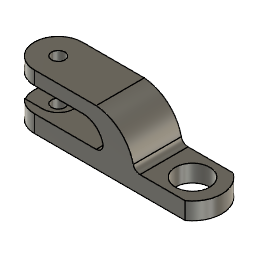
11_largage_moteur_manivelle (Autodesk Fusion 360 design; units mm, degrees)
Autodesk Fusion 360 part; units mm, degrees
note: some values were not read from the file. Set by a fixed rule: which sketch regions a step uses.
sketch "Esquisse2" plane through (0, 0, 0) normal (0, 0, 1) x (1, 0, 0)
  line L0 (0, 0) -> (34.1782, 0)
  line L1 (0, 14) -> (34.1782, 14)
  arc A0 (0, 14) -> (0, 0) centre (0, 7) ccw
  circle A1 centre (0, 7) radius 1.95
  circle A2 centre (39, 7) radius 5
  line L2 (39, 7) -> (46, 7) construction
  arc A3 (43.8218, 0) -> (43.8218, 14) centre (39, 7) ccw
  line L3 (34.1782, 14) -> (43.8218, 14)
  line L4 (34.1782, 0) -> (43.8218, 0)
  dimension "d10" = 3.9
  dimension "d15" = 17
  dimension "d16" = 39
  dimension "d17" = 10
  dimension "d18" = 14
  constraint coincident L0.start A0.end
  constraint horizontal L0
  constraint tangent L1 A0
  constraint tangent L0 A0
  constraint concentric A0 A1
  constraint coincident A2.centre L2.start
  constraint concentric A2 A3
  constraint parallel L1 L3
  constraint parallel L0 L4
  measures "d10" diameter of A1
  measures "d15" diameter of A3
  measures "d16" distance of A0.centre A2.centre
  measures "d17" diameter of A2
  measures "d18" distance of L0 L1
extrude "Extrusion1" add sketch "Esquisse2" along normal blind 16
sketch "Esquisse3" plane through (0, 0, 0) normal (0, 1, 0) x (1, 0, 0)
  line L0 (-7, 0) -> (-7, -5) construction
  line L1 (-7, -16.0714) -> (-7, -12.0714) construction
  line L2 (-7, -12.0714) -> (14.0533, -12.0714)
  arc A0 (18, -16) -> (28.7636, -6.5727) centre (17, -4) ccw
  line L3 (30.7174, -5) -> (48, -5)
  line L4 (48, -5) -> (48, -16)
  line L5 (18, -16) -> (48, -16)
  arc A1 (30.7174, -5) -> (28.7636, -6.5727) centre (30.7174, -7) ccw
  line L6 (18, -5) -> (-7, -5)
  line L7 (-7, -12.0714) -> (-7, -5)
  arc A2 (19.9387, -7.4912) -> (18, -5) centre (18, -7) ccw
  arc A3 (14.0533, -12.0714) -> (19.9387, -7.4912) centre (14.0533, -6) ccw
  point P0 (18, -12.0714)
  dimension "d21" = 5
  dimension "d22" = 4
  dimension "d23" = 25
  dimension "d25" = 2
  constraint vertical L0
  constraint vertical L1
  constraint perpendicular L1 L2
  constraint coincident P0 L2
  constraint horizontal L3
  constraint perpendicular L3 L4
  constraint perpendicular L4 L5
  constraint tangent L3 A1
  constraint tangent A0 A1
  constraint parallel L0 L7
  constraint tangent L6 A2
  constraint tangent A2 A3
  constraint tangent L2 A3
  measures "d21" distance of L0.start L0.end
  measures "d22" distance of L1.start L1.end
  measures "d23" distance of L1.end P0
  measures "d25" radius of A1
extrude "Extrusion2" cut sketch "Esquisse3" along normal blind 16 and the other way blind 2
sketch "Esquisse4" plane through (0, 0, 5) normal (0, 0, 1) x (-1, 0, 0)
  line L0 (-18, -14) -> (0, -14)
  arc A0 (0, -14) -> (0, 0) centre (0, -7) ccw
  line L1 (0, 0) -> (-18, 0)
  line L2 (-18, 0) -> (-18, -14)
  circle A1 centre (0, -7) radius 1.95
  line L3 (0, -14) -> (0, 0) construction
  line L4 (0, -11.6) -> (5.2764, -11.6)
  line L5 (0, -2.4) -> (5.2764, -2.4)
  arc A2 (0, -2.4) -> (0, -11.6) centre (0, -7) ccw
  dimension "d30" = 9.2
  constraint coincident L0.end A0.start
  constraint coincident A0.end L1.start
  constraint concentric A0 A2
  constraint coincident L3 L4.start
  constraint coincident A0 L4.end
  constraint tangent L4 A2
  constraint coincident L3 L5.start
  constraint coincident A0 L5.end
  constraint tangent L5 A2
  measures "d30" diameter of A2
extrude "Extrusion3" cut sketch "Esquisse4" against normal blind 1 contours A0 L4 L5 A2
extrude "Extrusion4" cut sketch "Esquisse4" along normal blind -1 and the other way blind -8 contours A0 L4 L5 A2
equation "d30 = 8 * 1.15 mm"
